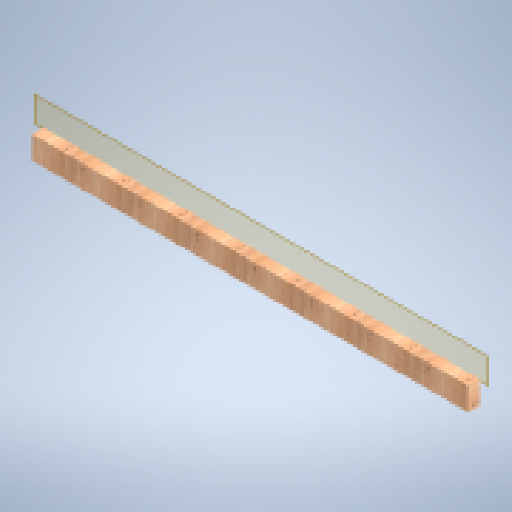
# Autodesk Inventor part: 2x4x76
Saved by Autodesk Inventor 2025 (Build 290162000, 162)
## iProperties
Created: 2024-09-08
Part Number: 2x4x76
Material: Wood (Birch)
Document SubType Name: Modeling
Designer: Win
Density: 0.55 g/cm^3
Appearance: Birch - Natural Polished
Author: Win
Autodesk Inventor part; units mm, degrees
ref_plane "YZ Plane" through (0, 0, 0) normal (1, 0, 0) x (0, 1, 0)
ref_plane "XZ Plane" through (0, 0, 0) normal (0, 1, 0) x (-1, 0, 0)
ref_plane "XY Plane" through (0, 0, 0) normal (0, 0, 1) x (1, 0, 0)
ref_plane "Work Plane1" through (0, 0, 0) normal (0, 0, 1) x (1, 0, 0)
sketch "Sketch1" plane through (0, 0, 0) normal (0, 0, 1) x (1, 0, 0)
  line L0 (0, 0) -> (0, -101.6) projected
  line L1 (0, 0) -> (-1828.8, 0) projected
  line L2 (-1828.8, 0) -> (-1828.8, -101.6) projected
  line L3 (0, -101.6) -> (-1828.8, -101.6) projected
  line L4 (50.8, -101.6) -> (0, -101.6) projected
  line L5 (50.8, 0) -> (50.8, -101.6) projected
  line L6 (-1828.8, -101.6) -> (-1879.6, -101.6) projected
  line L7 (-1828.8, 0) -> (-1828.8, -101.6) projected
  line L8 (-1879.6, -50.8) -> (-1879.6, -101.6) projected
  line L9 (-1879.6, -101.6) -> (50.8, -101.6)
  line L10 (50.8, -101.6) -> (50.8, -203.2)
  line L11 (50.8, -203.2) -> (-1879.6, -203.2)
  line L12 (-1879.6, -203.2) -> (-1879.6, -101.6)
  dimension "d0" = 101.6
  constraints: 8 end point, 2 parallel, 1 horizontal, 1 perpendicular
  measures "d0" distance of L9.end L10.end
extrude "Extrusion1" add sketch "Sketch1" along normal blind 50.8 contours L4 L10 L11 L12 L6 L3
body "Solid1"
